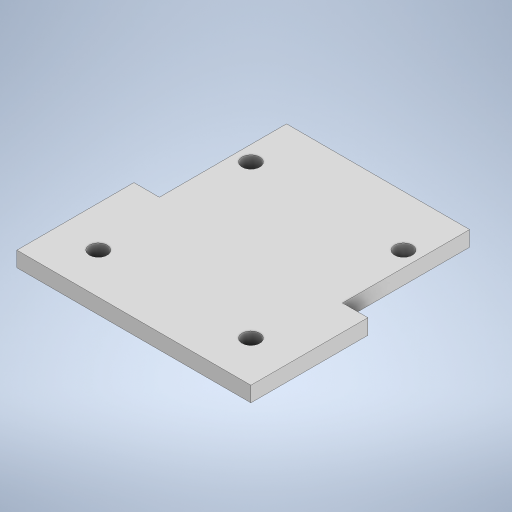
# Autodesk Inventor part: Metal Plate for Arm Clamp Thingy for Keaton because he Asked so here it is thanks
Saved by Autodesk Inventor 2023 (Build 270158000, 158)
## iProperties
Created: 2023-04-13
Part Number: Metal Plate for Arm Clamp Thingy for Keaton because he Asked so here it is thanks
Material: Generic
Document SubType Name: Sheet Metal
Designer: aidan
Density: 1 g/cm^3
Sheet Metal Rule: Default
Appearance: Default
Author: aidan
Autodesk Inventor part; units mm, degrees
ref_plane "YZ Plane" through (0, 0, 0) normal (1, 0, 0) x (0, 1, 0)
ref_plane "XZ Plane" through (0, 0, 0) normal (0, 1, 0) x (-1, 0, 0)
ref_plane "XY Plane" through (0, 0, 0) normal (0, 0, 1) x (1, 0, 0)
sketch "Sketch1" plane through (0, 0, 0) normal (0, 1, 0) x (-1, 0, 0)
  line L0 (37.125, 9.5155) -> (-8.875, 9.5155)
  line L1 (-8.875, 9.5155) -> (-8.875, -13.4845)
  line L2 (-8.875, -13.4845) -> (-3.875, -13.4845)
  line L3 (-3.875, -13.4845) -> (-3.875, -38.4845)
  line L4 (-3.875, -38.4845) -> (32.125, -38.4845)
  line L5 (32.125, -38.4845) -> (32.125, -13.4845)
  line L6 (32.125, -13.4845) -> (37.125, -13.4845)
  line L7 (37.125, -13.4845) -> (37.125, 9.5155)
  circle A0 centre (29.125, 1.5155) radius 1.75
  circle A1 centre (-0.875, 1.5155) radius 1.75
  circle A2 centre (-0.875, -28.4845) radius 1.75
  circle A3 centre (29.125, -28.4845) radius 1.75
  point P0 (0, 0)
  point P1 (14.125, -46.4845)
  dimension "d42" = 46
  dimension "d43" = 23
  dimension "d44" = 5
  dimension "d45" = 25
  dimension "d46" = 36
  dimension "d47" = 5
  constraints: 16 end point, 4 centre point, 3 perpendicular, 2 horizontal, 2 point on line, 1 vertical
  measures "d42" distance of L0.start L0.end
  measures "d43" distance of L0.end L1.end
  measures "d44" distance of L1.end L2.end
  measures "d45" distance of L2.end L3.end
  measures "d46" distance of L3.end L4.end
  measures "d47" distance of L5.end L6.end
extrude "Extrusion1" add sketch "Sketch1" along normal blind 3
equation "\"BendRadius\" = Thickness"
equation "\"BendReliefWidth\" = Thickness"
equation "\"BendReliefDepth\" = 0.5 * Thickness"
equation "\"CornerReliefSize\" = 4 * Thickness"
equation "\"MinimumRemnant\" = 2 * Thickness"
equation "\"TransitionRadius\" = BendRadius"
equation "\"JacobiRadiusSize\" = BendRadius"
equation "\"GapSize\" = Thickness"
equation "\"Thickness\" = 3.048"
body "Solid1"
